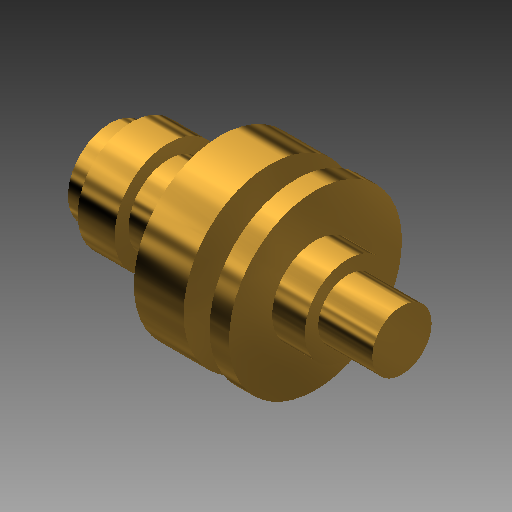
# Autodesk Inventor part: 403-10
Saved by Autodesk Inventor 2019 (Build 230136000, 136)
## iProperties
Company: Autodesk Inc.
Created: 2017-06-27
Part Number: 403-10
Material: Brass, Soft Yellow
Document SubType Name: Modeling
Designer: Autodesk Inc.
Mass: 2.26717 g
Surface Area: 4.32672 cm^2
Volume: 0.267671 cm^3
Density: 8.47 g/cm^3
Appearance: Brass - Satin
Author: Inventor
Autodesk Inventor part; units mm, degrees
ref_plane "YZ Plane" through (0, 0, 0) normal (1, 0, 0) x (0, 1, 0)
ref_plane "XZ Plane" through (0, 0, 0) normal (0, 1, 0) x (-1, 0, 0)
ref_plane "XY Plane" through (0, 0, 0) normal (0, 0, 1) x (1, 0, 0)
sketch "Sketch1" plane through (0, 0, 0) normal (0, 0, 1) x (1, 0, 0)
  line L0 (0, 0) -> (1, 0)
  line L1 (1, 0) -> (1, 1.95)
  line L2 (1, 1.95) -> (0, 1.95)
  line L3 (0, 1.95) -> (0, 0)
  line L4 (1, 0) -> (2.7, 0)
  line L5 (2.7, 0) -> (2.7, 2.5)
  line L6 (2.7, 2.5) -> (1, 2.5)
  line L7 (1, 2.5) -> (1, 0)
  line L8 (2.7, 0) -> (3.9, 0)
  line L9 (3.9, 0) -> (3.9, 1.85)
  line L10 (3.9, 1.85) -> (2.7, 1.85)
  line L11 (2.7, 1.85) -> (2.7, 0)
  line L12 (3.9, 0) -> (5.1, 0)
  line L13 (5.1, 0) -> (5.1, 2)
  line L14 (5.1, 2) -> (3.9, 2)
  line L15 (3.9, 2) -> (3.9, 0)
  line L16 (5.1, 0) -> (7.4, 0)
  line L17 (7.4, 0) -> (7.4, 4)
  line L18 (7.4, 4) -> (5.1, 4)
  line L19 (5.1, 4) -> (5.1, 0)
  line L20 (7.4, 0) -> (8.6, 0)
  line L21 (8.6, 0) -> (8.6, 2)
  line L22 (8.6, 2) -> (7.4, 2)
  line L23 (7.4, 2) -> (7.4, 0)
  line L24 (8.6, 0) -> (9.5, 0)
  line L25 (9.5, 0) -> (9.5, 4)
  line L26 (9.5, 4) -> (8.6, 4)
  line L27 (8.6, 4) -> (8.6, 0)
  line L28 (9.5, 0) -> (11, 0)
  line L29 (11, 0) -> (11, 2)
  line L30 (11, 2) -> (9.5, 2)
  line L31 (9.5, 2) -> (9.5, 0)
  line L32 (11, 0) -> (13.5, 0)
  line L33 (13.5, 0) -> (13.5, 1.375)
  line L34 (13.5, 1.375) -> (11, 1.375)
  line L35 (11, 1.375) -> (11, 0)
  dimension "d0" = 2.75
  dimension "d1" = 13.5
  dimension "d2" = 4
  dimension "d3" = 3.7
  dimension "d4" = 3.9
  dimension "d5" = 8
  dimension "d6" = 4
  dimension "d7" = 1
  dimension "d8" = 2.7
  dimension "d9" = 11
  dimension "d10" = 9.5
  dimension "d11" = 8.6
  dimension "d12" = 7.4
  dimension "d13" = 5.1
  dimension "d14" = 3.9
  dimension "d25" = 5
  constraints: 72 end point, 18 parallel, 9 horizontal, 9 perpendicular, 2 collinear
  measures "d0" diameter of L34 L32
  measures "d1" distance between parallel lines of L33 L3
  measures "d2" diameter of L30 L32
  measures "d3" diameter of L10 L0
  measures "d4" diameter of L2 L0
  measures "d5" diameter of L26 L32
  measures "d6" diameter of L22 L32
  measures "d7" distance of L1.end L2.end
  measures "d8" distance between parallel lines of L5 L3
  measures "d9" distance between parallel lines of L35 L3
  measures "d10" distance between parallel lines of L31 L3
  measures "d11" distance between parallel lines of L27 L3
  measures "d12" distance between parallel lines of L23 L3
  measures "d13" distance between parallel lines of L19 L3
  measures "d14" distance between parallel lines of L15 L3
  measures "d25" diameter of L6 L4
revolve "Revolution1" add sketch "Sketch1" angle 360 about axis through (0, 0, 0) along (1, 0, 0)
hole "Hole1" at (0, 0, 0) direction (1, 0, 0) diameter 1.567 depth 6.5 tip angle 118 counterbore diameter 2 counterbore depth 2 thread size "M2x0.4" class "6H" standard "ANSI Metric M Profile"
body "Solid1"
